Autodesk Fusion 360 part; units mm, degrees
(part 2 of 2)
  spline S309 degree 3 poles (23.5597, 49.4163) (23.5597, 48.0198) (23.5523, 46.8789) (23.5449, 46.8789) knots 0 0 0 0 1 1 1 1
  line L121 (13.051, 53.0019) -> (13.2066, 53.0834)
  spline S310 degree 3 poles (12.5176, 53.6316) (12.9213, 53.8539) (12.3139, 53.8428) (23.0448, 53.8428) knots 0 0 0 0 1 1 1 1
  line L122 (13.2066, 53.0834) -> (23.0004, 53.0945)
  line L123 (21.8558, 51.9536) -> (22.7077, 51.9536)
  spline S311 degree 3 poles (12.7954, 53.5724) (12.562, 53.4909) (12.3213, 53.2908) (12.2175, 53.0871) knots 0 0 0 0 1 1 1 1
  line L124 (23.5597, 51.9536) -> (23.5597, 49.4163)
  spline S312 degree 3 poles (22.5966, 34.4959) (22.4892, 34.5366) (22.3484, 34.6404) (22.1855, 34.7996) knots 0 0 0 0 1 1 1 1
  line L125 (23.0522, 44.4416) -> (22.7633, 45.4306)
  spline S313 degree 3 poles (23.0522, 46.027) (22.9041, 46.027) (22.7818, 46.0159) (22.7818, 45.9973) knots 0 0 0 0 1 1 1 1
  spline S314 degree 3 poles (12.2064, 52.2722) (12.3176, 52.0129) (22.0817, 35.1589) (22.2151, 34.9997) knots 0 0 0 0 1 1 1 1
  line L126 (23.5597, 51.9536) -> (23.5597, 49.4163)
  line L127 (22.7077, 51.9536) -> (23.5597, 51.9536)
  spline S315 degree 3 poles (23.5449, 46.8789) (23.5338, 46.8789) (23.1522, 47.3642) (22.6929, 47.9568) knots 0 0 0 0 1 1 1 1
  spline S316 degree 3 poles (21.9669, 45.9751) (21.9669, 45.7269) (22.4781, 43.7674) (22.5411, 43.7674) knots 0 0 0 0 1 1 1 1
  spline S317 degree 3 poles (23.4412, 35.3738) (23.3115, 35.2367) (23.1041, 35.1367) (22.9633, 35.1367) knots 0 0 0 0 1 1 1 1
  spline S318 degree 3 poles (24.5265, 45.4565) (24.5339, 45.4491) (24.9969, 45.4269) (25.5562, 45.4047) knots 0 0 0 0 1 1 1 1
  spline S319 degree 3 poles (23.0411, 53.639) (13.4881, 53.639) (12.9732, 53.6353) (12.7954, 53.5724) knots 0 0 0 0 1 1 1 1
  line L128 (22.6929, 47.9568) -> (21.8558, 49.031)
  spline S320 degree 3 poles (23.5449, 46.8789) (23.5338, 46.8789) (23.1522, 47.3642) (22.6929, 47.9568) knots 0 0 0 0 1 1 1 1
  spline S321 degree 3 poles (23.0411, 52.25) (17.8849, 52.25) (13.6696, 52.2389) (13.6696, 52.2277) knots 0 0 0 0 1 1 1 1
  spline S322 degree 3 poles (23.4041, 42.4376) (23.356, 42.4413) (22.6966, 42.5376) (21.9373, 42.6562) knots 0 0 0 0 1 1 1 1
  spline S323 degree 3 poles (24.9414, 43.2563) (24.0079, 43.2525) (23.1411, 43.2674) (22.9004, 43.2896) knots 0 0 0 0 1 1 1 1
  spline S324 degree 3 poles (22.7818, 45.9973) (22.7781, 45.9529) (23.3523, 44.0304) (23.3634, 44.0415) knots 0 0 0 0 1 1 1 1
  line L129 (23.0522, 44.4416) -> (22.7633, 45.4306)
  spline S325 degree 3 poles (23.0411, 53.639) (13.4881, 53.639) (12.9732, 53.6353) (12.7954, 53.5724) knots 0 0 0 0 1 1 1 1
  spline S326 degree 3 poles (20.4593, 46.1344) (20.663, 46.2011) (23.7079, 46.2048) (24.182, 46.1381) knots 0 0 0 0 1 1 1 1
  spline S327 degree 3 poles (24.9414, 43.2563) (24.0079, 43.2525) (23.1411, 43.2674) (22.9004, 43.2896) knots 0 0 0 0 1 1 1 1
  spline S328 degree 3 poles (33.0794, 53.8057) (33.5165, 53.7242) (33.861, 53.476) (34.0203, 53.139) knots 0 0 0 0 1 1 1 1
  spline S329 degree 3 poles (23.0337, 43.4341) (23.1708, 43.4192) (23.293, 43.4044) (23.3115, 43.4007) knots 0 0 0 0 1 1 1 1
  spline S330 degree 3 poles (23.4004, 34.5107) (23.1485, 34.4181) (22.8374, 34.4144) (22.5966, 34.4959) knots 0 0 0 0 1 1 1 1
  spline S331 degree 3 poles (23.0522, 46.027) (22.9041, 46.027) (22.7818, 46.0159) (22.7818, 45.9973) knots 0 0 0 0 1 1 1 1
  spline S332 degree 3 poles (23.0448, 53.8428) (29.5012, 53.8428) (32.9535, 53.8316) (33.0794, 53.8057) knots 0 0 0 0 1 1 1 1
  spline S333 degree 3 poles (23.4004, 34.5107) (23.1485, 34.4181) (22.8374, 34.4144) (22.5966, 34.4959) knots 0 0 0 0 1 1 1 1
  spline S334 degree 3 poles (28.4159, 43.823) (25.2192, 38.326) (23.5412, 35.4738) (23.4412, 35.3738) knots 0 0 0 0 1 1 1 1
  spline S335 degree 3 poles (23.7079, 34.9256) (23.8264, 35.0515) (25.2303, 37.437) (28.8307, 43.6267) knots 0 0 0 0 1 1 1 1
  spline S336 degree 3 poles (23.4412, 35.3738) (23.3115, 35.2367) (23.1041, 35.1367) (22.9633, 35.1367) knots 0 0 0 0 1 1 1 1
  spline S337 degree 3 poles (33.861, 52.3574) (34.0462, 52.8908) (33.8091, 53.3909) (33.2831, 53.5724) knots 0 0 0 0 1 1 1 1
  spline S338 degree 3 poles (28.4159, 43.823) (25.2192, 38.326) (23.5412, 35.4738) (23.4412, 35.3738) knots 0 0 0 0 1 1 1 1
  spline S339 degree 3 poles (22.5336, 35.3627) (22.3966, 35.5145) (12.7472, 52.2166) (12.7213, 52.3463) knots 0 0 0 0 1 1 1 1
  spline S340 degree 3 poles (32.9905, 53.013) (33.1202, 52.9538) (33.2165, 52.8797) (33.2646, 52.7982) knots 0 0 0 0 1 1 1 1
  line L130 (32.7942, 53.1019) -> (32.9905, 53.013)
  spline S341 degree 3 poles (33.2646, 52.7982) (33.3498, 52.6537) (33.3609, 52.413) (33.2868, 52.2389) knots 0 0 0 0 1 1 1 1
  spline S342 degree 3 poles (13.6696, 52.2277) (13.6696, 52.1685) (23.0596, 36.3628) (23.0819, 36.3887) knots 0 0 0 0 1 1 1 1
  line L131 (32.7942, 53.1019) -> (32.9905, 53.013)
  spline S343 degree 3 poles (12.2064, 52.2722) (12.3176, 52.0129) (22.0817, 35.1589) (22.2151, 34.9997) knots 0 0 0 0 1 1 1 1
  spline S344 degree 3 poles (34.0203, 53.139) (34.1203, 52.9204) (34.1203, 52.5278) (34.0166, 52.2685) knots 0 0 0 0 1 1 1 1
  spline S345 degree 3 poles (13.6696, 52.2277) (13.6696, 52.1685) (23.0596, 36.3628) (23.0819, 36.3887) knots 0 0 0 0 1 1 1 1
  spline S346 degree 3 poles (28.9826, 43.5452) (23.5523, 34.1959) (23.8486, 34.6774) (23.4004, 34.5107) knots 0 0 0 0 1 1 1 1
  spline S347 degree 3 poles (34.0203, 53.139) (34.1203, 52.9204) (34.1203, 52.5278) (34.0166, 52.2685) knots 0 0 0 0 1 1 1 1
  spline S348 degree 3 poles (28.9826, 43.5452) (23.5523, 34.1959) (23.8486, 34.6774) (23.4004, 34.5107) knots 0 0 0 0 1 1 1 1
  spline S349 degree 3 poles (23.0819, 36.3887) (23.093, 36.4035) (25.2006, 39.9707) (27.7602, 44.3156) knots 0 0 0 0 1 1 1 1
  spline S350 degree 3 poles (23.0819, 36.3887) (23.093, 36.4035) (25.2006, 39.9707) (27.7602, 44.3156) knots 0 0 0 0 1 1 1 1
  spline S351 degree 3 poles (23.3856, 34.6885) (23.4708, 34.7256) (23.6153, 34.833) (23.7079, 34.9256) knots 0 0 0 0 1 1 1 1
  spline S352 degree 3 poles (33.861, 52.3574) (34.0462, 52.8908) (33.8091, 53.3909) (33.2831, 53.5724) knots 0 0 0 0 1 1 1 1
  spline S353 degree 3 poles (22.9633, 35.1367) (22.9337, 35.1367) (22.8448, 35.1701) (22.7633, 35.2071) knots 0 0 0 0 1 1 1 1
  spline S354 degree 3 poles (33.2646, 52.7982) (33.3498, 52.6537) (33.3609, 52.413) (33.2868, 52.2389) knots 0 0 0 0 1 1 1 1
  spline S355 degree 3 poles (22.7929, 34.6144) (22.9485, 34.5774) (23.1967, 34.607) (23.3856, 34.6885) knots 0 0 0 0 1 1 1 1
  spline S356 degree 3 poles (32.9905, 53.013) (33.1202, 52.9538) (33.2165, 52.8797) (33.2646, 52.7982) knots 0 0 0 0 1 1 1 1
  spline S357 degree 3 poles (22.5336, 35.3627) (22.3966, 35.5145) (12.7472, 52.2166) (12.7213, 52.3463) knots 0 0 0 0 1 1 1 1
  spline S358 degree 3 poles (34.0166, 52.2685) (33.9795, 52.1648) (31.7126, 48.2384) (28.9826, 43.5452) knots 0 0 0 0 1 1 1 1
  spline S359 degree 3 poles (34.0166, 52.2685) (33.9795, 52.1648) (31.7126, 48.2384) (28.9826, 43.5452) knots 0 0 0 0 1 1 1 1
  spline S360 degree 3 poles (23.0448, 53.8428) (29.5012, 53.8428) (32.9535, 53.8316) (33.0794, 53.8057) knots 0 0 0 0 1 1 1 1
  spline S361 degree 3 poles (22.1855, 34.7996) (21.9558, 35.0293) (21.6669, 35.522) (17.0404, 43.5267) knots 0 0 0 0 1 1 1 1
  spline S362 degree 3 poles (23.3856, 34.6885) (23.4708, 34.7256) (23.6153, 34.833) (23.7079, 34.9256) knots 0 0 0 0 1 1 1 1
  spline S363 degree 3 poles (22.2151, 34.9997) (22.3521, 34.8293) (22.604, 34.6626) (22.7929, 34.6144) knots 0 0 0 0 1 1 1 1
  spline S364 degree 3 poles (33.0794, 53.8057) (33.5165, 53.7242) (33.861, 53.476) (34.0203, 53.139) knots 0 0 0 0 1 1 1 1
  spline S365 degree 3 poles (22.1855, 34.7996) (21.9558, 35.0293) (21.6669, 35.522) (17.0404, 43.5267) knots 0 0 0 0 1 1 1 1
  spline S366 degree 3 poles (27.7602, 44.3156) (30.3198, 48.6643) (32.4127, 52.224) (32.4127, 52.2352) knots 0 0 0 0 1 1 1 1
  spline S367 degree 3 poles (33.2831, 53.5724) (33.109, 53.6353) (32.5423, 53.639) (23.0411, 53.639) knots 0 0 0 0 1 1 1 1
  line L132 (82.4079, 16.7934) -> (79.8747, 16.5479)
  spline S368 degree 2 poles (79.8747, 16.5479) (79.6464, 17.8234) (78.9473, 18.4217) knots 0 0 0 1 1 1
  spline S369 degree 2 poles (78.9473, 18.4217) (78.2483, 19.02) (77.0609, 19.0203) knots 0 0 0 1 1 1
  spline S370 degree 2 poles (77.0609, 19.0203) (75.8031, 19.0207) (75.1652, 18.4888) knots 0 0 0 1 1 1
  spline S371 degree 2 poles (75.1652, 18.4888) (74.5274, 17.9568) (74.5272, 17.2444) knots 0 0 0 1 1 1
  spline S372 degree 2 poles (74.5272, 17.2444) (74.527, 16.787) (74.7952, 16.4659) knots 0 0 0 1 1 1
  spline S373 degree 2 poles (74.7952, 16.4659) (75.0634, 16.1448) (75.7318, 15.9071) knots 0 0 0 1 1 1
  spline S374 degree 2 poles (75.7318, 15.9071) (76.1891, 15.7486) (77.8162, 15.3435) knots 0 0 0 1 1 1
  spline S375 degree 2 poles (77.8162, 15.3435) (79.9094, 14.8239) (80.7535, 14.0673) knots 0 0 0 1 1 1
  spline S376 degree 2 poles (80.7535, 14.0673) (81.9406, 13.0026) (81.9402, 11.4722) knots 0 0 0 1 1 1
  spline S377 degree 2 poles (81.9402, 11.4722) (81.9399, 10.4871) (81.3811, 9.6297) knots 0 0 0 1 1 1
  spline S378 degree 2 poles (81.3811, 9.6297) (80.8223, 8.7722) (79.7711, 8.324) knots 0 0 0 1 1 1
  spline S379 degree 2 poles (79.7711, 8.324) (78.7199, 7.8757) (77.2334, 7.8762) knots 0 0 0 1 1 1
  spline S380 degree 2 poles (77.2334, 7.8762) (74.8058, 7.8769) (73.5791, 8.9416) knots 0 0 0 1 1 1
  spline S381 degree 2 poles (73.5791, 8.9416) (72.3524, 10.0062) (72.2914, 11.783) knots 0 0 0 1 1 1
  line L133 (72.2914, 11.783) -> (74.895, 11.8965)
  spline S382 degree 2 poles (74.895, 11.8965) (75.0618, 10.9025) (75.6114, 10.467) knots 0 0 0 1 1 1
  spline S383 degree 2 poles (75.6114, 10.467) (76.161, 10.0314) (77.2604, 10.0311) knots 0 0 0 1 1 1
  spline S384 degree 2 poles (77.2604, 10.0311) (78.3951, 10.0308) (79.0373, 10.4967) knots 0 0 0 1 1 1
  spline S385 degree 2 poles (79.0373, 10.4967) (79.4508, 10.7957) (79.4509, 11.297) knots 0 0 0 1 1 1
  spline S386 degree 2 poles (79.4509, 11.297) (79.4511, 11.7544) (79.0642, 12.08) knots 0 0 0 1 1 1
  spline S387 degree 2 poles (79.0642, 12.08) (78.5717, 12.4935) (76.672, 12.9427) knots 0 0 0 1 1 1
  spline S388 degree 2 poles (76.672, 12.9427) (74.7723, 13.3918) (73.8621, 13.8715) knots 0 0 0 1 1 1
  spline S389 degree 2 poles (73.8621, 13.8715) (72.9519, 14.3511) (72.4376, 15.1824) knots 0 0 0 1 1 1
  spline S390 degree 2 poles (72.4376, 15.1824) (71.9233, 16.0138) (71.9236, 17.2364) knots 0 0 0 1 1 1
  spline S391 degree 2 poles (71.9236, 17.2364) (71.924, 18.3446) (72.54, 19.312) knots 0 0 0 1 1 1
  spline S392 degree 2 poles (72.54, 19.312) (73.156, 20.2793) (74.2819, 20.7495) knots 0 0 0 1 1 1
  spline S393 degree 2 poles (74.2819, 20.7495) (75.4079, 21.2198) (77.0879, 21.2193) knots 0 0 0 1 1 1
  spline S394 degree 2 poles (77.0879, 21.2193) (79.5331, 21.2185) (80.8433, 20.0879) knots 0 0 0 1 1 1
  spline S395 degree 2 poles (80.8433, 20.0879) (82.1535, 18.9572) (82.4079, 16.7934) knots 0 0 0 1 1 1
  line L134 (69.7171, 20.9928) -> (69.7132, 8.0984)
  line L135 (69.7132, 8.0984) -> (67.1096, 8.0991)
  line L136 (67.1096, 8.0991) -> (67.1112, 13.1742)
  line L137 (67.1112, 13.1742) -> (62.0097, 13.1758)
  line L138 (62.0097, 13.1758) -> (62.0082, 8.1007)
  line L139 (62.0082, 8.1007) -> (59.4046, 8.1015)
  line L140 (59.4046, 8.1015) -> (59.4085, 20.9959)
  line L141 (59.4085, 20.9959) -> (62.0121, 20.9951)
  line L142 (62.0121, 20.9951) -> (62.0104, 15.3571)
  line L143 (62.0104, 15.3571) -> (67.1118, 15.3556)
  line L144 (67.1118, 15.3556) -> (67.1136, 20.9936)
  line L145 (67.1136, 20.9936) -> (69.7171, 20.9928)
  line L146 (45.0804, 21.0003) -> (47.9126, 20.9994)
  line L147 (47.9126, 20.9994) -> (49.0376, 18.0701)
  line L148 (49.0376, 18.0701) -> (54.1918, 18.0686)
  line L149 (54.1918, 18.0686) -> (55.257, 20.9972)
  line L150 (55.257, 20.9972) -> (58.0188, 20.9964)
  line L151 (58.0188, 20.9964) -> (52.9926, 8.1034)
  line L152 (52.9926, 8.1034) -> (50.2395, 8.1043)
  line L153 (50.2395, 8.1043) -> (45.0804, 21.0003)
  line L154 (49.8725, 15.8973) -> (51.6478, 11.112)
  line L155 (51.6478, 11.112) -> (53.3908, 15.8963)
  line L156 (53.3908, 15.8963) -> (49.8725, 15.8973)
  line L157 (44.6758, 21.0004) -> (44.6719, 8.106)
  line L158 (44.6719, 8.106) -> (39.1922, 8.1076)
  spline S396 degree 2 poles (39.1922, 8.1076) (37.1252, 8.1082) (36.1886, 8.456) knots 0 0 0 1 1 1
  spline S397 degree 2 poles (36.1886, 8.456) (35.2519, 8.8037) (34.6893, 9.6922) knots 0 0 0 1 1 1
  spline S398 degree 2 poles (34.6893, 9.6922) (34.1266, 10.5807) (34.127, 11.7242) knots 0 0 0 1 1 1
  spline S399 degree 2 poles (34.127, 11.7242) (34.1274, 13.1755) (34.9809, 14.1207) knots 0 0 0 1 1 1
  spline S400 degree 2 poles (34.9809, 14.1207) (35.8344, 15.066) (37.532, 15.3118) knots 0 0 0 1 1 1
  spline S401 degree 2 poles (37.532, 15.3118) (36.6878, 15.8046) (36.1382, 16.3941) knots 0 0 0 1 1 1
  spline S402 degree 2 poles (36.1382, 16.3941) (35.5887, 16.9835) (34.6568, 18.4879) knots 0 0 0 1 1 1
  line L159 (34.6568, 18.4879) -> (33.0831, 21.0039)
  line L160 (33.0831, 21.0039) -> (36.1968, 21.003)
  line L161 (36.1968, 21.003) -> (38.0782, 18.1966)
  spline S403 degree 2 poles (38.0782, 18.1966) (39.0804, 16.6922) (39.4497, 16.3007) knots 0 0 0 1 1 1
  spline S404 degree 2 poles (39.4497, 16.3007) (39.819, 15.9092) (40.2324, 15.7639) knots 0 0 0 1 1 1
  spline S405 degree 2 poles (40.2324, 15.7639) (40.6457, 15.6187) (41.5429, 15.6184) knots 0 0 0 1 1 1
  line L162 (41.5429, 15.6184) -> (42.0706, 15.6182)
  line L163 (42.0706, 15.6182) -> (42.0723, 21.0012)
  line L164 (42.0723, 21.0012) -> (44.6758, 21.0004)
  line L165 (42.07, 13.5601) -> (40.1438, 13.5606)
  spline S406 degree 2 poles (40.1438, 13.5606) (38.2703, 13.5612) (37.8041, 13.403) knots 0 0 0 1 1 1
  spline S407 degree 2 poles (37.8041, 13.403) (37.3379, 13.2448) (37.0739, 12.8579) knots 0 0 0 1 1 1
  spline S408 degree 2 poles (37.0739, 12.8579) (36.8099, 12.471) (36.8097, 11.8905) knots 0 0 0 1 1 1
  spline S409 degree 2 poles (36.8097, 11.8905) (36.8095, 11.2396) (37.1568, 10.8393) knots 0 0 0 1 1 1
  spline S410 degree 2 poles (37.1568, 10.8393) (37.5041, 10.439) (38.1374, 10.3332) knots 0 0 0 1 1 1
  spline S411 degree 2 poles (38.1374, 10.3332) (38.454, 10.2892) (40.0372, 10.2887) knots 0 0 0 1 1 1
  line L166 (40.0372, 10.2887) -> (42.069, 10.2881)
  line L167 (42.069, 10.2881) -> (42.07, 13.5601)
  line L168 (31.667, 21.0043) -> (31.6631, 8.1099)
  line L169 (31.6631, 8.1099) -> (27.4852, 8.1112)
  spline S412 degree 2 poles (27.4852, 8.1112) (25.1103, 8.1119) (24.3891, 8.3056) knots 0 0 0 1 1 1
  spline S413 degree 2 poles (24.3891, 8.3056) (23.281, 8.5962) (22.5336, 9.5684) knots 0 0 0 1 1 1
  spline S414 degree 2 poles (22.5336, 9.5684) (21.7863, 10.5405) (21.7868, 12.0797) knots 0 0 0 1 1 1
  spline S415 degree 2 poles (21.7868, 12.0797) (21.7871, 13.2672) (22.2184, 14.0762) knots 0 0 0 1 1 1
  spline S416 degree 2 poles (22.2184, 14.0762) (22.6496, 14.8853) (23.3138, 15.3469) knots 0 0 0 1 1 1
  spline S417 degree 2 poles (23.3138, 15.3469) (23.978, 15.8084) (24.6641, 15.9578) knots 0 0 0 1 1 1
  spline S418 degree 2 poles (24.6641, 15.9578) (25.5965, 16.1422) (27.3645, 16.1416) knots 0 0 0 1 1 1
  line L170 (27.3645, 16.1416) -> (29.062, 16.1411)
  line L171 (29.062, 16.1411) -> (29.0635, 21.0051)
  line L172 (29.0635, 21.0051) -> (31.667, 21.0043)
  line L173 (29.0602, 10.292) -> (29.0614, 13.951)
  line L174 (29.0614, 13.951) -> (27.6365, 13.9514)
  spline S419 degree 2 poles (27.6365, 13.9514) (26.0972, 13.9519) (25.5782, 13.7498) knots 0 0 0 1 1 1
  spline S420 degree 2 poles (25.5782, 13.7498) (25.0592, 13.5476) (24.7644, 13.1167) knots 0 0 0 1 1 1
  spline S421 degree 2 poles (24.7644, 13.1167) (24.4696, 12.6858) (24.4695, 12.1141) knots 0 0 0 1 1 1
  spline S422 degree 2 poles (24.4695, 12.1141) (24.4692, 11.4105) (24.8825, 10.953) knots 0 0 0 1 1 1
  spline S423 degree 2 poles (24.8825, 10.953) (25.2958, 10.4955) (25.929, 10.3809) knots 0 0 0 1 1 1
  spline S424 degree 2 poles (25.929, 10.3809) (26.3952, 10.2928) (27.8025, 10.2924) knots 0 0 0 1 1 1
  line L175 (27.8025, 10.2924) -> (29.0602, 10.292)
  line L176 (20.3017, 16.8123) -> (17.7685, 16.5668)
  spline S425 degree 2 poles (17.7685, 16.5668) (17.5402, 17.8422) (16.8411, 18.4405) knots 0 0 0 1 1 1
  spline S426 degree 2 poles (16.8411, 18.4405) (16.1421, 19.0388) (14.9546, 19.0392) knots 0 0 0 1 1 1
  spline S427 degree 2 poles (14.9546, 19.0392) (13.6969, 19.0396) (13.059, 18.5076) knots 0 0 0 1 1 1
  spline S428 degree 2 poles (13.059, 18.5076) (12.4212, 17.9757) (12.4209, 17.2632) knots 0 0 0 1 1 1
  spline S429 degree 2 poles (12.4209, 17.2632) (12.4208, 16.8059) (12.689, 16.4847) knots 0 0 0 1 1 1
  spline S430 degree 2 poles (12.689, 16.4847) (12.9571, 16.1636) (13.6255, 15.9259) knots 0 0 0 1 1 1
  spline S431 degree 2 poles (13.6255, 15.9259) (14.0829, 15.7675) (15.7099, 15.3624) knots 0 0 0 1 1 1
  spline S432 degree 2 poles (15.7099, 15.3624) (17.8032, 14.8428) (18.6473, 14.0861) knots 0 0 0 1 1 1
  spline S433 degree 2 poles (18.6473, 14.0861) (19.8344, 13.0215) (19.8339, 11.491) knots 0 0 0 1 1 1
  spline S434 degree 2 poles (19.8339, 11.491) (19.8336, 10.5059) (19.2749, 9.6485) knots 0 0 0 1 1 1
  spline S435 degree 2 poles (19.2749, 9.6485) (18.7161, 8.7911) (17.6649, 8.3428) knots 0 0 0 1 1 1
  spline S436 degree 2 poles (17.6649, 8.3428) (16.6136, 7.8946) (15.1272, 7.895) knots 0 0 0 1 1 1
  spline S437 degree 2 poles (15.1272, 7.895) (12.6996, 7.8958) (11.4729, 8.9604) knots 0 0 0 1 1 1
  spline S438 degree 2 poles (11.4729, 8.9604) (10.2462, 10.0251) (10.1852, 11.8018) knots 0 0 0 1 1 1
  line L177 (10.1852, 11.8018) -> (12.7887, 11.9154)
  spline S439 degree 2 poles (12.7887, 11.9154) (12.9556, 10.9214) (13.5052, 10.4858) knots 0 0 0 1 1 1
  spline S440 degree 2 poles (13.5052, 10.4858) (14.0547, 10.0503) (15.1542, 10.05) knots 0 0 0 1 1 1
  spline S441 degree 2 poles (15.1542, 10.05) (16.2889, 10.0496) (16.9311, 10.5156) knots 0 0 0 1 1 1
  spline S442 degree 2 poles (16.9311, 10.5156) (17.3446, 10.8145) (17.3447, 11.3159) knots 0 0 0 1 1 1
  spline S443 degree 2 poles (17.3447, 11.3159) (17.3449, 11.7732) (16.9579, 12.0988) knots 0 0 0 1 1 1
  spline S444 degree 2 poles (16.9579, 12.0988) (16.4655, 12.5123) (14.5658, 12.9615) knots 0 0 0 1 1 1
  spline S445 degree 2 poles (14.5658, 12.9615) (12.6661, 13.4107) (11.7558, 13.8903) knots 0 0 0 1 1 1
  spline S446 degree 2 poles (11.7558, 13.8903) (10.8456, 14.3699) (10.3313, 15.2013) knots 0 0 0 1 1 1
  spline S447 degree 2 poles (10.3313, 15.2013) (9.8171, 16.0326) (9.8174, 17.2552) knots 0 0 0 1 1 1
  spline S448 degree 2 poles (9.8174, 17.2552) (9.8178, 18.3635) (10.4338, 19.3308) knots 0 0 0 1 1 1
  spline S449 degree 2 poles (10.4338, 19.3308) (11.0497, 20.2982) (12.1757, 20.7684) knots 0 0 0 1 1 1
  spline S450 degree 2 poles (12.1757, 20.7684) (13.3017, 21.2386) (14.9817, 21.2381) knots 0 0 0 1 1 1
  spline S451 degree 2 poles (14.9817, 21.2381) (17.4269, 21.2374) (18.7371, 20.1067) knots 0 0 0 1 1 1
  spline S452 degree 2 poles (18.7371, 20.1067) (20.0473, 18.9761) (20.3017, 16.8123) knots 0 0 0 1 1 1
  constraint midpoint L4 L71.start
  constraint midpoint L6 L71.end
  constraint symmetric S0.start L71 S306.start
  constraint symmetric S0.end L71 S306.end
  constraint symmetric S0 L71 S312
  constraint symmetric S1.end L71 S248.start
  constraint symmetric S1 L71 S361
  constraint symmetric S2.end L71 S248.end
  constraint symmetric S2 L71 S282
  constraint symmetric S3.end L71 S237.start
  constraint symmetric S3 L71 S283
  constraint symmetric S4.end L71 S237.end
  constraint symmetric S4 L71 S249
  constraint symmetric S5.end L71 S308.end
  constraint symmetric S5 L71 S310
  constraint symmetric S6.end L71 S328.start
  constraint symmetric S6 L71 S360
  constraint symmetric S7.end L71 S328.end
  constraint symmetric S7 L71 S328
  constraint symmetric S8.end L71 S344.end
  constraint symmetric S8 L71 S347
  constraint symmetric S9.end L71 S346.start
  constraint symmetric S9 L71 S359
  constraint symmetric S10.end L71 S330.start
  constraint symmetric S10 L71 S346
  constraint symmetric S11 L71 S333
  constraint symmetric S12.start L71 S268.end
  constraint symmetric S12.end L71 S300.start
  constraint symmetric S12 L71 S362
  constraint symmetric S13.end L71 S266.start
  constraint symmetric S13 L71 S335
  constraint symmetric S14.end L71 S266.end
  constraint symmetric S14 L71 S266
  constraint symmetric S15.end L71 S267.start
  constraint symmetric S15 L71 S352
  constraint symmetric S16.end L71 S267.end
  constraint symmetric S16 L71 S367
  constraint symmetric S17.end L71 S285.start
  constraint symmetric S17 L71 S325
  constraint symmetric S18.end L71 S234.start
  constraint symmetric S18 L71 S285
  constraint symmetric S19.end L71 S234.end
  constraint symmetric S19 L71 S234
  constraint symmetric S20.end L71 S294.start
  constraint symmetric S20 L71 S314
  constraint symmetric S21.end L71 S268.start
  constraint symmetric S21 L71 S363
  constraint symmetric S22 L71 S355
  constraint symmetric S23.start L71 S291.end
  constraint symmetric S23.end L71 S295.end
  constraint symmetric S23 L71 S299
  constraint symmetric S24.end L71 S275.start
  constraint symmetric S24 L71 S357
  constraint symmetric S25.end L71 L92.start
  constraint symmetric S25 L71 S297
  constraint symmetric L8.end L71 L92.end
  constraint symmetric L9.end L71 L72.start
  constraint symmetric L10.end L71 L72.end
  constraint symmetric L11.end L71 S340.start
  constraint symmetric S26.end L71 S340.end
  constraint symmetric S26 L71 S356
  constraint symmetric S27.end L71 S186.start
  constraint symmetric S27 L71 S341
  constraint symmetric S28.end L71 S186.end
  constraint symmetric S28 L71 S290
  constraint symmetric S29.end L71 S317.start
  constraint symmetric S29 L71 S338
  constraint symmetric S30.end L71 S291.start
  constraint symmetric S30 L71 S336
  constraint symmetric S31 L71 S353
  constraint symmetric S32.start L71 S265.start
  constraint symmetric S32.end L71 S184.start
  constraint symmetric S32 L71 S265
  constraint symmetric S33.end L71 S184.end
  constraint symmetric S33 L71 S184
  constraint symmetric S34.end L71 S292.end
  constraint symmetric S34 L71 S292
  constraint symmetric S35.end L71 S342.end
  constraint symmetric S35 L71 S345
  constraint symmetric S36 L71 S349
  constraint symmetric S37.start L71 S255.start
  constraint symmetric S37.end L71 S225.start
  constraint symmetric S37 L71 S255
  constraint symmetric S38.end L71 S225.end
  constraint symmetric S38 L71 S236
  constraint symmetric S39.end L71 S243.end
  constraint symmetric S39 L71 S243
  constraint symmetric S40.end L71 L97.start
  constraint symmetric S40 L71 S276
  constraint symmetric L12.end L71 L94.start
  constraint symmetric L13.end L71 L94.end
  constraint symmetric L14.end L71 L96.end
  constraint symmetric L15.end L71 L99.end
  constraint symmetric S41.end L71 S254.start
  constraint symmetric S41 L71 S288
  constraint symmetric S42.end L71 S254.end
  constraint symmetric S42 L71 S254
  constraint symmetric S43.end L71 S286.start
  constraint symmetric S43 L71 S326
  constraint symmetric S44.end L71 S204.start
  constraint symmetric S44 L71 S302
  constraint symmetric S45.end L71 S204.end
  constraint symmetric S45 L71 S215
  constraint symmetric S46.end L71 S213.start
  constraint symmetric S46 L71 S214
  constraint symmetric S47.end L71 S213.end
  constraint symmetric S47 L71 S218
  constraint symmetric S48.end L71 S273.end
  constraint symmetric S48 L71 S273
  constraint symmetric S49.end L71 S190.start
  constraint symmetric S49 L71 S318
  constraint symmetric S50.end L71 S189.start
  constraint symmetric S50 L71 S252
  constraint symmetric S51.end L71 S189.end
  constraint symmetric S51 L71 S253
  constraint symmetric L16.end L71 L80.end
  constraint symmetric L17.end L71 S203.start
  constraint symmetric S52.end L71 S203.end
  constraint symmetric S52 L71 S226
  constraint symmetric S53.end L71 L86.start
  constraint symmetric S53 L71 S258
  constraint symmetric L18.end L71 L86.end
  constraint symmetric L19.end L71 L91.end
  constraint symmetric S54.end L71 L73.start
  constraint symmetric S54 L71 S279
  constraint symmetric L20.end L71 L73.end
  constraint symmetric L21.end L71 S188.start
  constraint symmetric S55.end L71 S188.end
  constraint symmetric S55 L71 S188
  constraint symmetric S56.end L71 S202.start
  constraint symmetric S56 L71 S257
  constraint symmetric S57.end L71 S202.end
  constraint symmetric S57 L71 S244
  constraint symmetric S58.end L71 S193.start
  constraint symmetric S58 L71 S211
  constraint symmetric S59.end L71 S193.end
  constraint symmetric S59 L71 S262
  constraint symmetric S60.end L71 S227.start
  constraint symmetric S60 L71 S323
  constraint symmetric S61.end L71 S227.end
  constraint symmetric S61 L71 S278
  constraint symmetric S62.end L71 S232.end
  constraint symmetric S62 L71 S233
  constraint symmetric S63.end L71 S201.start
  constraint symmetric S63 L71 S305
  constraint symmetric S64.end L71 S201.end
  constraint symmetric S64 L71 S201
  constraint symmetric S65 L71 S322
  constraint symmetric S66.start L71 S191.end
  constraint symmetric S66.end L71 S235.end
  constraint symmetric S66 L71 S250
  constraint symmetric L22.end L71 L102.start
  constraint symmetric L23.end L71 S206.start
  constraint symmetric S67.end L71 S206.end
  constraint symmetric S67 L71 S228
  constraint symmetric S68.end L71 S209.end
  constraint symmetric S68 L71 S209
  constraint symmetric S69.end L71 S191.start
  constraint symmetric S69 L71 S329
  constraint symmetric S70 L71 S205
  constraint symmetric S71.start L71 S208.end
  constraint symmetric S71.end L71 L74.start
  constraint symmetric S71 L71 S247
  constraint symmetric L24.end L71 L74.end
  constraint symmetric L25.end L71 L82.end
  constraint symmetric S72.end L71 L78.start
  constraint symmetric S72 L71 S241
  constraint symmetric L26.end L71 L78.end
  constraint symmetric L27.end L71 S208.start
  constraint symmetric S73 L71 S208
  constraint symmetric S74.start L71 S216.end
  constraint symmetric S74.end L71 S198.start
  constraint symmetric S74 L71 S260
  constraint symmetric S75.end L71 S192.start
  constraint symmetric S75 L71 S200
  constraint symmetric S76.end L71 S192.end
  constraint symmetric S76 L71 S192
  constraint symmetric S77.end L71 S216.start
  constraint symmetric S77 L71 S238
  constraint symmetric S78 L71 S216
  constraint symmetric L28.start L71 S259.end
  constraint symmetric L28.end L71 L106.end
  constraint symmetric L29.end L71 S272.start
  constraint symmetric S79.end L71 S272.end
  constraint symmetric S79 L71 S274
  constraint symmetric S80.end L71 S259.start
  constraint symmetric S80 L71 S281
  constraint symmetric S81 L71 S263
  constraint symmetric L30.start L71 S187.end
  constraint symmetric L30.end L71 L77.start
  constraint symmetric L31.end L71 L77.end
  constraint symmetric S82.end L71 S307.start
  constraint symmetric S82 L71 S313
  constraint symmetric S83.end L71 S187.start
  constraint symmetric S83 L71 S324
  constraint symmetric S84 L71 S187
  constraint symmetric S85.start L71 S196.end
  constraint symmetric S85.end L71 S197.start
  constraint symmetric S85 L71 S229
  constraint symmetric S86.end L71 S194.start
  constraint symmetric S86 L71 S197
  constraint symmetric S87.end L71 S194.end
  constraint symmetric S87 L71 S194
  constraint symmetric S88.end L71 S196.start
  constraint symmetric S88 L71 S224
  constraint symmetric S89 L71 S269
  constraint symmetric L32.start L71 L115.start
  constraint symmetric L32.end L71 L110.start
  constraint symmetric L33.end L71 L110.end
  constraint symmetric L34.end L71 L113.end
  constraint symmetric L35.end L71 L114.end
  constraint symmetric L36.end L71 L120.end
  constraint symmetric L37.end L71 S298.start
  constraint symmetric S90.end L71 S298.end
  constraint symmetric S90 L71 S298
  constraint symmetric S91 L71 S315
  constraint symmetric S92 L71 S344
  constraint symmetric S93 L71 S366
  constraint symmetric S94 L71 S358
  constraint symmetric S95 L71 S340
  constraint symmetric S96 L71 S337
  constraint symmetric S97 L71 S232
  constraint symmetric S98 L71 S304
  constraint symmetric S99 L71 S196
  constraint symmetric S100 L71 S301
  constraint symmetric S101 L71 S213
  constraint symmetric S102 L71 S242
  constraint symmetric S103 L71 S261
  constraint symmetric S104 L71 S277
  constraint symmetric S105 L71 S220
  constraint symmetric S106 L71 S307
  constraint symmetric S107 L71 S239
  constraint symmetric S108 L71 S231
  constraint symmetric S109 L71 S259
  constraint symmetric S110 L71 S207
  constraint symmetric S111 L71 S199
  constraint symmetric S112 L71 S198
  constraint symmetric S113 L71 S287
  constraint symmetric S114 L71 S189
  constraint symmetric S115 L71 S296
  constraint symmetric S116 L71 S309
  constraint symmetric S117 L71 S321
  constraint symmetric S118 L71 S320
  constraint symmetric S119 L71 S230
  constraint symmetric S120 L71 S185
  constraint symmetric S121 L71 S327
  constraint symmetric S122 L71 S217
  constraint symmetric S123 L71 S225
  constraint symmetric S124 L71 S291
  constraint symmetric S125 L71 S295
  constraint symmetric S126 L71 S332
  constraint symmetric S127 L71 S339
  constraint symmetric S128 L71 S343
  constraint symmetric S129 L71 S342
  constraint symmetric S130 L71 S365
  constraint symmetric S131 L71 S319
  constraint symmetric S132 L71 S308
  constraint symmetric S133 L71 S334
  constraint symmetric S134 L71 S267
  constraint symmetric S135 L71 S351
  constraint symmetric S136 L71 S350
  constraint symmetric S137 L71 S268
  constraint symmetric S138 L71 S300
  constraint symmetric S139 L71 S251
  constraint symmetric S140 L71 S193
  constraint symmetric S141 L71 S202
  constraint symmetric S142 L71 S223
  constraint symmetric S143 L71 S190
  constraint symmetric S144 L71 S284
  constraint symmetric S145 L71 S235
  constraint symmetric S146 L71 S264
  constraint symmetric S147 L71 S246
  constraint symmetric S148 L71 S219
  constraint symmetric S149 L71 S303
  constraint symmetric S150 L71 S272
  constraint symmetric S151 L71 S227
  constraint symmetric S152 L71 S210
  constraint symmetric S153 L71 S316
  constraint symmetric S154 L71 S271
  constraint symmetric S155 L71 S240
  constraint symmetric S156 L71 S206
  constraint symmetric S157 L71 S203
  constraint symmetric S158 L71 S204
  constraint symmetric S159 L71 S245
  constraint symmetric S160 L71 S195
  constraint symmetric S161 L71 S331
  constraint symmetric S162 L71 S191
  constraint symmetric S163 L71 S270
  constraint symmetric S164 L71 S293
  constraint symmetric S165 L71 S222
  constraint symmetric S166 L71 S221
  constraint symmetric S167 L71 S212
  constraint symmetric S168 L71 S286
  constraint symmetric S169 L71 S311
  constraint symmetric S170 L71 S280
  constraint symmetric S171 L71 S237
  constraint symmetric S172 L71 S248
  constraint symmetric S173 L71 S275
  constraint symmetric S174 L71 S306
  constraint symmetric S175 L71 S256
  constraint symmetric S176 L71 S294
  constraint symmetric S177 L71 S330
  constraint symmetric S178 L71 S317
  constraint symmetric S179 L71 S348
  constraint symmetric S180 L71 S364
  constraint symmetric S181 L71 S354
  constraint symmetric S182 L71 S289
  constraint symmetric S183 L71 S186
extrude "Extrude4" add sketch "Sketch4" along normal blind 2 contours L71 L146 L147 L148 L149 L150 L151 L152 L153 | L71 L146 L153 | S0 S1 S2 S3 S4 S5 S6 S7 S8 S9 S10 S11 S92 S94 S126 S130 S132 S171 S172 S174 S175 S177 S179 S180 | S12 S13 S14 S15 S16 S17 S18 S19 S20 S21 S22 S96 S128 S131 S134 S135 S137 S138 S169 S170 S176 S182 | S37 S38 S39 S40 L12 L13 L14 L15 S41 S42 S43 S44 S45 S46 S47 S48 S49 S50 S51 L16 L17 S52 S53 L18 L19 S54 L20 L21 S55 S56 S57 S58 S59 S60 S61 S62 S63 S64 S65 S97 S98 S100 L40 S101 S102 S103 S104 L44 S105 S108 S110 L47 S113 S114 L48 S115 S121 S122 S123 S140 S141 S143 S144 L53 L54 L55 S146 S148 L57 S151 S157 S158 L60 S159 S163 S164 L65 S168 | L32 L33 L34 L35 L36 L37 S90 S91 L38 L39 L41 L42 L43 S116 S118 L59 | S188 S189 S190 L73 S193 L75 S201 S202 S203 S204 L79 S207 S211 L80 L81 S213 S214 L84 S215 L86 S217 L88 S218 S219 S220 L91 S225 S226 L93 S227 L94 L95 S231 S232 S233 S236 L96 S242 L97 S243 S244 S245 L98 L99 L100 L101 S252 S253 S254 S255 S257 L103 S258 L104 S261 S262 S264 S270 S273 S276 S277 S278 S279 S284 S286 S287 S288 S293 S296 S301 S302 S304 S305 S318 S322 S323 S326 S327 | S234 S266 S267 S268 S280 S285 S289 S294 S300 S311 S314 S319 S325 S335 S337 S343 S351 S352 S355 S362 S363 S367 | S237 S248 S249 S256 S282 S283 S306 S308 S310 S312 S328 S330 S332 S333 S344 S346 S347 S348 S358 S359 S360 S361 S364 S365 | L110 L113 L114 L115 L116 L117 S298 L120 S309 L123 L124 L126 L127 S315 L128 S320 | L132 S368 S369 S370 S371 S372 S373 S374 S375 S376 S377 S378 S379 S380 S381 L133 S382 S383 S384 S385 S386 S387 S388 S389 S390 S391 S392 S393 S394 S395 | L134 L135 L136 L137 L138 L139 L140 L141 L142 L143 L144 L145 | L157 L158 S396 S397 S398 S399 S400 S401 S402 L159 L160 L161 S403 S404 S405 L162 L163 L164 | L168 L169 S412 S413 S414 S415 S416 S417 S418 L170 L171 L172 | L176 S425 S426 S427 S428 S429 S430 S431 S432 S433 S434 S435 S436 S437 S438 L177 S439 S440 S441 S442 S443 S444 S445 S446 S447 S448 S449 S450 S451 S452
extrude "Extrude5" add sketch "Sketch3" along normal blind 2 contours L5 A2 L6 L11 | L6 A3 L7 L8 | A0 L4 L7 L9 | L4 A1 L5 L10
extrude "Extrude6" add sketch "Sketch3" along normal blind 1.6 contours L6 L7 L8 L15 | L5 L6 L11 L12 | L4 L7 L9 L14 | L4 L5 L10 L13
extrude "Extrude7" add sketch "Sketch3" along normal blind 1.2 contours L0 L12 L15 L20 L21 | L2 L13 L14 L18 L19 | L14 L15 L16 | L12 L13 L17
extrude "Extrude8" add sketch "Sketch3" along normal blind 0.8 contours L15 L16 L21 L23 | L12 L17 L20 L21 L25 | L14 L16 L19 L22 | L13 L17 L18 L19 L24
extrude "Extrude9" add sketch "Sketch3" along normal blind 0.4 contours L22 L23 L27 | L24 L25 L26
equation "d12 = d11"
